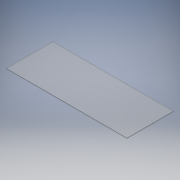
# Autodesk Inventor part: Scheibe
Saved by Autodesk Inventor 2016 SP2 (Build 200236200, 236)
## iProperties
Created: 2018-06-21
Part Number: Scheibe
Material: PMMA-Kunststoff
Document SubType Name: Modeling
Designer: Nils
Density: 1.188 g/cm^3
Appearance: Polycarbonat - klar
Author: Nils
Autodesk Inventor part; units mm, degrees
ref_plane "YZ Plane" through (0, 0, 0) normal (1, 0, 0) x (0, 1, 0)
ref_plane "XZ Plane" through (0, 0, 0) normal (0, 1, 0) x (-1, 0, 0)
ref_plane "XY Plane" through (0, 0, 0) normal (0, 0, 1) x (1, 0, 0)
sketch "Skizze1" plane through (0, 0, 0) normal (0, 0, 1) x (1, 0, 0)
  line L0 (0, 0) -> (397.6, 0)
  line L1 (397.6, 0) -> (397.6, 153.5)
  line L2 (397.6, 153.5) -> (0, 153.5)
  line L3 (0, 153.5) -> (0, 0)
  dimension "d0" = 397.6
  dimension "d1" = 153.5
  constraints: 8 end point, 2 parallel, 1 horizontal, 1 perpendicular
  measures "d0" distance of L2.end L1.end
  measures "d1" distance of L1.end L0.end
extrude "Extrusion1" add sketch "Skizze1" along normal blind 2
